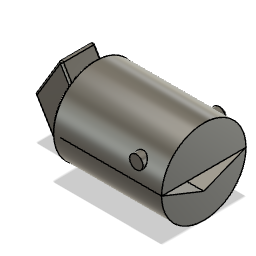
Shape 4 (Autodesk Fusion 360 design; units mm, degrees)
Autodesk Fusion 360 part; units mm, degrees
sketch "Sketch1" plane through (0, 0, 0) normal (1, 0, 0) x (0, 0, -1)
  circle A0 centre (0, 0) radius 25
  constraint coincident A0.centre origin
extrude "Extrude1" add sketch "Sketch1" along normal blind 60 makes body 1
sketch "Sketch2" plane through (0, 0, 0) normal (0, 0, 1) x (1, 0, 0)
  line L0 (0, 0) -> (-15, 25)
  line L1 (-15, 25) -> (-30, 0)
  line L2 (-30, 0) -> (-15, -25)
  line L3 (-15, -25) -> (0, 0)
  constraint coincident L0.start L3.end
  constraint parallel L0 L2
  constraint parallel L1 L3
extrude "Extrude2" add sketch "Sketch2" along normal blind 10 and the other way blind 10 separate body makes body 2
sketch "Sketch3" plane through (0, 0, 0) normal (0, 0, 1) x (1, 0, 0)
  circle A0 centre (45, 10) radius 4
  dimension "d7" = 8
  measures "d7" diameter of A0
extrude "Extrude3" add sketch "Sketch3" along normal mid plane 50 bodies 1
extrude "Extrude4" add 1 faces at (0, -1.242, 6.7759) along direction (-1, 0, 0) blind 5 on bodies 1 bodies 1 2
sketch "Sketch4" plane through (0, 0, 0) normal (1, 0, 0) x (0, 0, -1)
  line L0 (-25, 0) -> (0, -10)
  line L1 (0, -10) -> (25, 0)
  line L2 (25, 0) -> (-25, 0)
  constraint coincident L0 L2.end
  constraint horizontal L2
extrude "Extrude5" cut sketch "Sketch4" along normal blind 60 bodies 1
fillet "Fillet1" radius 1 5 edges at (-10, 16.6667, 10) (-22.5, 12.5, 10) (-22.5, -12.5, 10) (-10, -16.6667, 10) (-5, 9.0404, 23.3082) on bodies 1
fillet "Fillet2" radius 1 3 edges at (41.2707, 11.4465, -25) (-22.5, 12.5, -10) (-22.5, -12.5, -10) on bodies 1
fillet "Fillet3" radius 1 7 edges at (-29.6584, 0, -9.7071) (-30, 0, 0) (-29.6584, 0, 9.7071) (-15, -24.4307, 9.7071) (-15, -25, 0) (-14.8292, -24.7154, -9.7071) (-9.7085, -16.1808, -10) on bodies 1
fillet "Fillet4" radius 1 4 edges at (-15, 24.4307, 9.7071) (-15, 25, 0) (-14.8292, 24.7154, -9.7071) (-9.7085, 16.1808, -10) on bodies 1
